Magnet-Klauber v4 (Autodesk Fusion 360 archive; units mm, degrees)
design "Gleitgestell"
Autodesk Fusion 360 part; units mm, degrees
(part 1 of 2)
sketch "Skizze1" plane through (0, 0, 0) normal (0, 0, 1) x (1, 0, 0)
  line L0 (0, 0) -> (18.25, 0) construction
  line L1 (18.25, 0) -> (30.25, 0)
  line L2 (30.25, 0) -> (30.25, 22)
  line L3 (30.25, 22) -> (18.25, 22)
  line L4 (18.25, 22) -> (18.25, 0)
  circle A0 centre (26.25, 14.5) radius 1.5
  line L5 (0, 25) -> (0, 0) construction
  line L6 (-18.25, 22) -> (-18.25, 0)
  line L7 (-18.25, 0) -> (-30.25, 0)
  line L8 (-30.25, 0) -> (-30.25, 22)
  circle A1 centre (-26.25, 14.5) radius 1.5
  line L9 (-30.25, 22) -> (-18.25, 22)
  dimension "d8" = 12
  dimension "d9" = 22
  dimension "d10" = 3
  dimension "d11" = 4
  dimension "d12" = 7.5
  dimension "d25" = 26.25
  constraint coincident L0.start L5.end
  constraint horizontal L0
  constraint horizontal L1
  constraint vertical L2
  constraint horizontal L3
  constraint vertical L4
  constraint vertical L5
  constraint symmetric L0.end L5 L6.end
  constraint symmetric L1.end L5 L7.end
  constraint symmetric L2.end L5 L8.end
  constraint symmetric L3.end L5 L6.start
  constraint symmetric A0 L5 A1
  measures "d8" distance of L0.end L1.end
  measures "d9" distance of L0.end L3.end
  measures "d10" diameter of A0
  measures "d11" distance of L2 A0.centre
  measures "d12" distance of L3 A0.centre
  measures "d25" distance of A0.centre L5
extrude "Extrusion1" add sketch "Skizze1" against normal blind 3 makes body 1 at (24.8054, 4.3459, 0) makes body 2 at (-24.8054, 4.3459, 0)
sketch "Skizze2" plane through (0, 0, -3) normal (0, 0, -1) x (1, 0, 0)
  circle A0 centre (-26.25, -14.5) radius 1.5
  line L0 (-30.25, 0) -> (-30.25, -22)
  line L1 (-30.25, -22) -> (-18.25, -22)
  line L2 (-18.25, -22) -> (-18.25, 0)
  line L3 (-18.25, 0) -> (-30.25, 0)
  circle A1 centre (26.25, -14.5) radius 1.5
  line L4 (18.25, 0) -> (30.25, 0)
  line L5 (30.25, 0) -> (30.25, -22)
  line L6 (30.25, -22) -> (18.25, -22)
  line L7 (18.25, -22) -> (18.25, 0)
  circle A2 centre (-26.25, -14.5) radius 1.5
  line L8 (-18.25, 0) -> (-30.25, 0)
  line L9 (-18.25, -22) -> (-18.25, 0)
  line L10 (-30.25, -22) -> (-18.25, -22)
  line L11 (-30.25, 0) -> (-30.25, -22)
  line L12 (-30.25, 1) -> (-18.25, 1)
  line L13 (-18.25, 1) -> (-18.25, -22)
  line L14 (-30.25, -22) -> (-30.25, 1)
  line L15 (0, 0) -> (0, -27) construction
  line L16 (18.25, -22) -> (30.25, -22)
  line L17 (30.25, 1) -> (18.25, 1)
  dimension "d27" = 1
  constraint horizontal L12
  constraint vertical L13
  constraint vertical L14
  constraint coincident L11 L12.start
  constraint coincident L15.start origin
  constraint vertical L15
  constraint symmetric L12.start L15 L17.start
  constraint symmetric L12.end L15 L17.end
  constraint symmetric L1.end L15 L6.end
  constraint symmetric L0.end L15 L5.end
  constraint coincident L1.end L2.start
  constraint coincident L0.end L1.start
  measures "d27" distance of L8 L12
extrude "Extrusion2" add sketch "Skizze2" along normal blind 29 contours A0 A2 | L0 L1 L2 L3 L8 L9 L10 L11 L13 L14 | A1 | L4 L5 L6 L7 L16 bodies 1 2
thread "Gewinde1" "ISO Metric profile 3.0 M3x0.5 6H" major diameter 3.086 minor diameter 2.529 pitch 0.5 angle 60 resizes the face on face at (-24.7519, 14.4252, -2) on face at (27.7481, 14.4252, -2) on bodies 1 2
sketch "Skizze3" plane through (30.25, 0, 0) normal (1, 0, 0) x (0, 1, 0)
  line L0 (22, 0) -> (0, 0)
  line L1 (0, 0) -> (0, -32)
  line L2 (0, -32) -> (22, -32)
  line L3 (22, -32) -> (22, 0)
  circle A0 centre (9.5, -22) radius 6.5
  dimension "d19" = 13
  dimension "d24" = 22
  dimension "d28" = 9.5
  measures "d19" diameter of A0
  measures "d24" distance of L0 A0.centre
  measures "d28" distance of L1 A0.centre
extrude "Extrusion3" cut sketch "Skizze3" against normal blind 93 contours A0 bodies 1 2

design "2020_T-Nut"
Autodesk Fusion 360 part; units mm, degrees
sketch "Skizze1" plane through (0, 0, 0) normal (1, 0, 0) x (0, 1, 0)
  line L0 (0, 0) -> (3.5, 0)
  line L1 (5, 1.5) -> (5, 3.3)
  line L2 (5, 3.3) -> (2.5, 3.3)
  line L3 (2.5, 3.3) -> (2.5, 5)
  line L4 (3.5, 0) -> (5, 1.5)
  line L5 (0, 5) -> (0, 0) construction
  line L6 (-5, 1.5) -> (-5, 3.3)
  line L7 (-5, 3.3) -> (-2.5, 3.3)
  line L8 (0, 0) -> (-3.5, 0)
  line L9 (-3.5, 0) -> (-5, 1.5)
  line L10 (-2.5, 3.3) -> (-2.5, 5)
  line L11 (-2.5, 5) -> (2.5, 5)
  point P0 (5, 0)
  point P1 (-5, 0)
  point P2 (0, 0)
  point P3 (0, 0)
  dimension "d1" = 5
  dimension "d3" = 2.5
  dimension "d4" = 3.3
  dimension "d5" = 1.5
  dimension "d6" = 1.5
  constraint coincident P3 P2
  constraint horizontal L0
  constraint perpendicular L0 L1
  constraint perpendicular L1 L2
  constraint perpendicular L2 L3
  constraint coincident P0 L0
  constraint coincident P0 L1
  constraint perpendicular L0 L5
  constraint symmetric P3 L5 P2
  constraint symmetric P0 L5 P1
  constraint symmetric L1.end L5 L6.end
  constraint symmetric L2.end L5 L7.end
  constraint symmetric L3.end L5 L10.end
  constraint symmetric L0.end L5 L8.end
  constraint symmetric L1.start L5 L6.start
  measures "d1" distance of P3 P0
  measures "d3" distance of L1.end L2.end
  measures "d4" distance of L0 L2
  measures "d5" distance of P0 L0.end
  measures "d6" distance of P0 L1.start
extrude "Extrusion1" add sketch "Skizze1" along normal blind 11.5
sketch "Skizze2" plane through (0, 0, 5) normal (0, 0, 1) x (-1, 0, 0)
  line L0 (0, 0) -> (0, 2.5)
  line L1 (0, 2.5) -> (-11.5, 2.5)
  line L2 (-11.5, -2.5) -> (0, -2.5)
  circle A0 centre (-5.75, 0) radius 2
  line L3 (-11.5, 2.5) -> (-11.5, 0)
  line L4 (0, -2.5) -> (0, 0)
  line L5 (0, 0) -> (-11.5, 0)
  line L6 (-11.5, 0) -> (-11.5, -2.5)
  dimension "d9" = 4
  measures "d9" diameter of A0
extrude "Extrusion2" cut sketch "Skizze2" against normal blind 5.5 contours A0 L5 | A0 L5
thread "Gewinde1" "ISO Metric profile 4.0 M4x0.7 6H" major diameter 4.1095 minor diameter 3.332 pitch 0.7 angle 60 resizes the face on face at (7.7401, 0.1991, 1.6667)

design "Riemen"
Autodesk Fusion 360 part; units mm, degrees
sketch "Skizze1" plane through (0, 0, 0) normal (0, 0, 1) x (1, 0, 0)
  line L0 (-200, 5) -> (0, 5)
  line L1 (0, -5) -> (-200, -5)
  line L2 (0, -6) -> (-200, -6)
  line L3 (-200, 6) -> (0, 6)
  line L4 (-200, 5) -> (-200, -5) construction
  arc A0 (-200, 6) -> (-200, -6) centre (-200, 0) ccw
  arc A1 (-200, 5) -> (-200, -5) centre (-200, 0) ccw
  line L5 (0, -10) -> (0, 7.5) construction
  circle A2 centre (-1, -5) radius 0.5
  circle A3 centre (-3.0202, -5) radius 0.5
  circle A4 centre (-5.0404, -5) radius 0.5
  circle A5 centre (-7.0606, -5) radius 0.5
  circle A6 centre (-9.0808, -5) radius 0.5
  circle A7 centre (-11.101, -5) radius 0.5
  circle A8 centre (-13.1212, -5) radius 0.5
  circle A9 centre (-15.1414, -5) radius 0.5
  circle A10 centre (-17.1616, -5) radius 0.5
  circle A11 centre (-19.1818, -5) radius 0.5
  circle A12 centre (-21.202, -5) radius 0.5
  circle A13 centre (-23.2222, -5) radius 0.5
  circle A14 centre (-25.2424, -5) radius 0.5
  circle A15 centre (-27.2626, -5) radius 0.5
  circle A16 centre (-29.2828, -5) radius 0.5
  circle A17 centre (-31.303, -5) radius 0.5
  circle A18 centre (-33.3232, -5) radius 0.5
  circle A19 centre (-35.3434, -5) radius 0.5
  circle A20 centre (-37.3636, -5) radius 0.5
  circle A21 centre (-39.3838, -5) radius 0.5
  circle A22 centre (-41.404, -5) radius 0.5
  circle A23 centre (-43.4242, -5) radius 0.5
  circle A24 centre (-45.4444, -5) radius 0.5
  circle A25 centre (-47.4646, -5) radius 0.5
  circle A26 centre (-49.4848, -5) radius 0.5
  circle A27 centre (-51.5051, -5) radius 0.5
  circle A28 centre (-53.5253, -5) radius 0.5
  circle A29 centre (-55.5455, -5) radius 0.5
  circle A30 centre (-57.5657, -5) radius 0.5
  circle A31 centre (-59.5859, -5) radius 0.5
  circle A32 centre (-61.6061, -5) radius 0.5
  circle A33 centre (-63.6263, -5) radius 0.5
  circle A34 centre (-65.6465, -5) radius 0.5
  circle A35 centre (-67.6667, -5) radius 0.5
  circle A36 centre (-69.6869, -5) radius 0.5
  circle A37 centre (-71.7071, -5) radius 0.5
  circle A38 centre (-73.7273, -5) radius 0.5
  circle A39 centre (-75.7475, -5) radius 0.5
  circle A40 centre (-77.7677, -5) radius 0.5
  circle A41 centre (-79.7879, -5) radius 0.5
  circle A42 centre (-81.8081, -5) radius 0.5
  circle A43 centre (-83.8283, -5) radius 0.5
  circle A44 centre (-85.8485, -5) radius 0.5
  circle A45 centre (-87.8687, -5) radius 0.5
  circle A46 centre (-89.8889, -5) radius 0.5
  circle A47 centre (-91.9091, -5) radius 0.5
  circle A48 centre (-93.9293, -5) radius 0.5
  circle A49 centre (-95.9495, -5) radius 0.5
  circle A50 centre (-97.9697, -5) radius 0.5
  circle A51 centre (-99.9899, -5) radius 0.5
  circle A52 centre (-102.0101, -5) radius 0.5
  circle A53 centre (-104.0303, -5) radius 0.5
  circle A54 centre (-106.0505, -5) radius 0.5
  circle A55 centre (-108.0707, -5) radius 0.5
  circle A56 centre (-110.0909, -5) radius 0.5
  circle A57 centre (-112.1111, -5) radius 0.5
  circle A58 centre (-114.1313, -5) radius 0.5
  circle A59 centre (-116.1515, -5) radius 0.5
  circle A60 centre (-118.1717, -5) radius 0.5
  circle A61 centre (-120.1919, -5) radius 0.5
  circle A62 centre (-122.2121, -5) radius 0.5
  circle A63 centre (-124.2323, -5) radius 0.5
  circle A64 centre (-126.2525, -5) radius 0.5
  circle A65 centre (-128.2727, -5) radius 0.5
  circle A66 centre (-130.2929, -5) radius 0.5
  circle A67 centre (-132.3131, -5) radius 0.5
  circle A68 centre (-134.3333, -5) radius 0.5
  circle A69 centre (-136.3535, -5) radius 0.5
  circle A70 centre (-138.3737, -5) radius 0.5
  circle A71 centre (-140.3939, -5) radius 0.5
  circle A72 centre (-142.4141, -5) radius 0.5
  circle A73 centre (-144.4343, -5) radius 0.5
  circle A74 centre (-146.4545, -5) radius 0.5
  circle A75 centre (-148.4747, -5) radius 0.5
  circle A76 centre (-150.4949, -5) radius 0.5
  circle A77 centre (-152.5152, -5) radius 0.5
  circle A78 centre (-154.5354, -5) radius 0.5
  circle A79 centre (-156.5556, -5) radius 0.5
  circle A80 centre (-158.5758, -5) radius 0.5
  circle A81 centre (-160.596, -5) radius 0.5
  circle A82 centre (-162.6162, -5) radius 0.5
  circle A83 centre (-164.6364, -5) radius 0.5
  circle A84 centre (-166.6566, -5) radius 0.5
  circle A85 centre (-168.6768, -5) radius 0.5
  circle A86 centre (-170.697, -5) radius 0.5
  circle A87 centre (-172.7172, -5) radius 0.5
  circle A88 centre (-174.7374, -5) radius 0.5
  circle A89 centre (-176.7576, -5) radius 0.5
  circle A90 centre (-178.7778, -5) radius 0.5
  circle A91 centre (-180.798, -5) radius 0.5
  circle A92 centre (-182.8182, -5) radius 0.5
  circle A93 centre (-184.8384, -5) radius 0.5
  circle A94 centre (-186.8586, -5) radius 0.5
  circle A95 centre (-188.8788, -5) radius 0.5
  circle A96 centre (-190.899, -5) radius 0.5
  circle A97 centre (-192.9192, -5) radius 0.5
  circle A98 centre (-194.9394, -5) radius 0.5
  circle A99 centre (-196.9596, -5) radius 0.5
  circle A100 centre (-198.9798, -5) radius 0.5
  circle A101 centre (-205, 0) radius 0.5
  circle A102 centre (-201.5035, 4.7686) radius 0.5
  circle A103 centre (-203.324, 3.7351) radius 0.5
  circle A104 centre (-204.5618, 2.047) radius 0.5
  circle A105 centre (-204.5618, -2.047) radius 0.5
  circle A106 centre (-203.324, -3.7351) radius 0.5
  circle A107 centre (-201.5035, -4.7686) radius 0.5
  circle A108 centre (-1, 5) radius 0.5
  circle A109 centre (-3.0204, 5) radius 0.5
  circle A110 centre (-5.0408, 5) radius 0.5
  circle A111 centre (-7.0612, 5) radius 0.5
  circle A112 centre (-9.0816, 5) radius 0.5
  circle A113 centre (-11.102, 5) radius 0.5
  circle A114 centre (-13.1224, 5) radius 0.5
  circle A115 centre (-15.1429, 5) radius 0.5
  circle A116 centre (-17.1633, 5) radius 0.5
  circle A117 centre (-19.1837, 5) radius 0.5
  circle A118 centre (-21.2041, 5) radius 0.5
  circle A119 centre (-23.2245, 5) radius 0.5
  circle A120 centre (-25.2449, 5) radius 0.5
  circle A121 centre (-27.2653, 5) radius 0.5
  circle A122 centre (-29.2857, 5) radius 0.5
  circle A123 centre (-31.3061, 5) radius 0.5
  circle A124 centre (-33.3265, 5) radius 0.5
  circle A125 centre (-35.3469, 5) radius 0.5
  circle A126 centre (-37.3673, 5) radius 0.5
  circle A127 centre (-39.3878, 5) radius 0.5
  circle A128 centre (-41.4082, 5) radius 0.5
  circle A129 centre (-43.4286, 5) radius 0.5
  circle A130 centre (-45.449, 5) radius 0.5
  circle A131 centre (-47.4694, 5) radius 0.5
  circle A132 centre (-49.4898, 5) radius 0.5
  circle A133 centre (-51.5102, 5) radius 0.5
  circle A134 centre (-53.5306, 5) radius 0.5
  circle A135 centre (-55.551, 5) radius 0.5
  circle A136 centre (-57.5714, 5) radius 0.5
  circle A137 centre (-59.5918, 5) radius 0.5
  circle A138 centre (-61.6122, 5) radius 0.5
  circle A139 centre (-63.6327, 5) radius 0.5
  circle A140 centre (-65.6531, 5) radius 0.5
  circle A141 centre (-67.6735, 5) radius 0.5
  circle A142 centre (-69.6939, 5) radius 0.5
  circle A143 centre (-71.7143, 5) radius 0.5
  circle A144 centre (-73.7347, 5) radius 0.5
  circle A145 centre (-75.7551, 5) radius 0.5
  circle A146 centre (-77.7755, 5) radius 0.5
  circle A147 centre (-79.7959, 5) radius 0.5
  circle A148 centre (-81.8163, 5) radius 0.5
  circle A149 centre (-83.8367, 5) radius 0.5
  circle A150 centre (-85.8571, 5) radius 0.5
  circle A151 centre (-87.8776, 5) radius 0.5
  circle A152 centre (-89.898, 5) radius 0.5
  circle A153 centre (-91.9184, 5) radius 0.5
  circle A154 centre (-93.9388, 5) radius 0.5
  circle A155 centre (-95.9592, 5) radius 0.5
  circle A156 centre (-97.9796, 5) radius 0.5
  circle A157 centre (-100, 5) radius 0.5
  circle A158 centre (-102.0204, 5) radius 0.5
  circle A159 centre (-104.0408, 5) radius 0.5
  circle A160 centre (-106.0612, 5) radius 0.5
  circle A161 centre (-108.0816, 5) radius 0.5
  circle A162 centre (-110.102, 5) radius 0.5
  circle A163 centre (-112.1224, 5) radius 0.5
  circle A164 centre (-114.1429, 5) radius 0.5
  circle A165 centre (-116.1633, 5) radius 0.5
  circle A166 centre (-118.1837, 5) radius 0.5
  circle A167 centre (-120.2041, 5) radius 0.5
  circle A168 centre (-122.2245, 5) radius 0.5
  circle A169 centre (-124.2449, 5) radius 0.5
  circle A170 centre (-126.2653, 5) radius 0.5
  circle A171 centre (-128.2857, 5) radius 0.5
  circle A172 centre (-130.3061, 5) radius 0.5
  circle A173 centre (-132.3265, 5) radius 0.5
  circle A174 centre (-134.3469, 5) radius 0.5
  circle A175 centre (-136.3673, 5) radius 0.5
  circle A176 centre (-138.3878, 5) radius 0.5
  circle A177 centre (-140.4082, 5) radius 0.5
  circle A178 centre (-142.4286, 5) radius 0.5
  circle A179 centre (-144.449, 5) radius 0.5
  circle A180 centre (-146.4694, 5) radius 0.5
  circle A181 centre (-148.4898, 5) radius 0.5
  circle A182 centre (-150.5102, 5) radius 0.5
  circle A183 centre (-152.5306, 5) radius 0.5
  circle A184 centre (-154.551, 5) radius 0.5
  circle A185 centre (-156.5714, 5) radius 0.5
  circle A186 centre (-158.5918, 5) radius 0.5
  circle A187 centre (-160.6122, 5) radius 0.5
  circle A188 centre (-162.6327, 5) radius 0.5
  circle A189 centre (-164.6531, 5) radius 0.5
  circle A190 centre (-166.6735, 5) radius 0.5
  circle A191 centre (-168.6939, 5) radius 0.5
  circle A192 centre (-170.7143, 5) radius 0.5
  circle A193 centre (-172.7347, 5) radius 0.5
  circle A194 centre (-174.7551, 5) radius 0.5
  circle A195 centre (-176.7755, 5) radius 0.5
  circle A196 centre (-178.7959, 5) radius 0.5
  circle A197 centre (-180.8163, 5) radius 0.5
  circle A198 centre (-182.8367, 5) radius 0.5
  circle A199 centre (-184.8571, 5) radius 0.5
  circle A200 centre (-186.8776, 5) radius 0.5
  circle A201 centre (-188.898, 5) radius 0.5
  circle A202 centre (-190.9184, 5) radius 0.5
  circle A203 centre (-192.9388, 5) radius 0.5
  circle A204 centre (-194.9592, 5) radius 0.5
  circle A205 centre (-196.9796, 5) radius 0.5
  circle A206 centre (-199, 5) radius 0.5
  line L6 (200, 5) -> (0, 5)
  circle A207 centre (13.1224, 5) radius 0.5
  circle A208 centre (25.2449, 5) radius 0.5
  circle A209 centre (67.6735, 5) radius 0.5
  circle A210 centre (89.8889, -5) radius 0.5
  circle A211 centre (158.5918, 5) radius 0.5
  circle A212 centre (118.1717, -5) radius 0.5
  circle A213 centre (73.7347, 5) radius 0.5
  circle A214 centre (19.1818, -5) radius 0.5
  circle A215 centre (29.2857, 5) radius 0.5
  circle A216 centre (5.0408, 5) radius 0.5
  circle A217 centre (162.6327, 5) radius 0.5
  circle A218 centre (128.2857, 5) radius 0.5
  circle A219 centre (43.4242, -5) radius 0.5
  circle A220 centre (116.1633, 5) radius 0.5
  circle A221 centre (23.2222, -5) radius 0.5
  circle A222 centre (75.7475, -5) radius 0.5
  circle A223 centre (172.7172, -5) radius 0.5
  circle A224 centre (53.5306, 5) radius 0.5
  circle A225 centre (31.3061, 5) radius 0.5
  circle A226 centre (95.9495, -5) radius 0.5
  circle A227 centre (87.8776, 5) radius 0.5
  line L7 (200, 6) -> (0, 6)
  line L8 (0, -5) -> (200, -5)
  line L9 (0, -6) -> (200, -6)
  circle A228 centre (19.1837, 5) radius 0.5
  circle A229 centre (168.6939, 5) radius 0.5
  circle A230 centre (102.0101, -5) radius 0.5
  circle A231 centre (71.7071, -5) radius 0.5
  circle A232 centre (63.6263, -5) radius 0.5
  circle A233 centre (114.1313, -5) radius 0.5
  circle A234 centre (51.5051, -5) radius 0.5
  circle A235 centre (27.2653, 5) radius 0.5
  circle A236 centre (106.0612, 5) radius 0.5
  circle A237 centre (164.6364, -5) radius 0.5
  circle A238 centre (7.0606, -5) radius 0.5
  circle A239 centre (81.8163, 5) radius 0.5
  circle A240 centre (21.2041, 5) radius 0.5
  circle A241 centre (170.697, -5) radius 0.5
  circle A242 centre (79.7879, -5) radius 0.5
  circle A243 centre (49.4848, -5) radius 0.5
  circle A244 centre (67.6667, -5) radius 0.5
  circle A245 centre (23.2245, 5) radius 0.5
  circle A246 centre (122.2121, -5) radius 0.5
  circle A247 centre (160.596, -5) radius 0.5
  circle A248 centre (126.2525, -5) radius 0.5
  circle A249 centre (174.7551, 5) radius 0.5
  circle A250 centre (122.2245, 5) radius 0.5
  circle A251 centre (162.6162, -5) radius 0.5
  circle A252 centre (37.3673, 5) radius 0.5
  circle A253 centre (97.9796, 5) radius 0.5
  circle A254 centre (1, 5) radius 0.5
  circle A255 centre (17.1616, -5) radius 0.5
  circle A256 centre (33.3265, 5) radius 0.5
  circle A257 centre (104.0408, 5) radius 0.5
  circle A258 centre (95.9592, 5) radius 0.5
  circle A259 centre (65.6465, -5) radius 0.5
  circle A260 centre (172.7347, 5) radius 0.5
  circle A261 centre (13.1212, -5) radius 0.5
  circle A262 centre (3.0202, -5) radius 0.5
  circle A263 centre (93.9293, -5) radius 0.5
  circle A264 centre (75.7551, 5) radius 0.5
  circle A265 centre (63.6327, 5) radius 0.5
  circle A266 centre (180.798, -5) radius 0.5
  circle A267 centre (15.1414, -5) radius 0.5
  circle A268 centre (1, -5) radius 0.5
  circle A269 centre (126.2653, 5) radius 0.5
  circle A270 centre (57.5714, 5) radius 0.5
  circle A271 centre (108.0816, 5) radius 0.5
  circle A272 centre (49.4898, 5) radius 0.5
  circle A273 centre (35.3434, -5) radius 0.5
  circle A274 centre (83.8367, 5) radius 0.5
  circle A275 centre (124.2449, 5) radius 0.5
  circle A276 centre (85.8485, -5) radius 0.5
  circle A277 centre (166.6566, -5) radius 0.5
  circle A278 centre (69.6869, -5) radius 0.5
  circle A279 centre (45.449, 5) radius 0.5
  circle A280 centre (53.5253, -5) radius 0.5
  circle A281 centre (47.4646, -5) radius 0.5
  circle A282 centre (65.6531, 5) radius 0.5
  circle A283 centre (158.5758, -5) radius 0.5
  circle A284 centre (91.9184, 5) radius 0.5
  circle A285 centre (118.1837, 5) radius 0.5
  circle A286 centre (178.7959, 5) radius 0.5
  circle A287 centre (102.0204, 5) radius 0.5
  circle A288 centre (128.2727, -5) radius 0.5
  circle A289 centre (168.6768, -5) radius 0.5
  circle A290 centre (39.3838, -5) radius 0.5
  circle A291 centre (17.1633, 5) radius 0.5
  circle A292 centre (124.2323, -5) radius 0.5
  circle A293 centre (27.2626, -5) radius 0.5
  circle A294 centre (184.8571, 5) radius 0.5
  circle A295 centre (104.0303, -5) radius 0.5
  circle A296 centre (110.102, 5) radius 0.5
  circle A297 centre (99.9899, -5) radius 0.5
  circle A298 centre (156.5556, -5) radius 0.5
  circle A299 centre (41.4082, 5) radius 0.5
  circle A300 centre (97.9697, -5) radius 0.5
  circle A301 centre (110.0909, -5) radius 0.5
  circle A302 centre (73.7273, -5) radius 0.5
  circle A303 centre (37.3636, -5) radius 0.5
  circle A304 centre (116.1515, -5) radius 0.5
  circle A305 centre (5.0404, -5) radius 0.5
  circle A306 centre (45.4444, -5) radius 0.5
  circle A307 centre (77.7755, 5) radius 0.5
  circle A308 centre (55.5455, -5) radius 0.5
  circle A309 centre (39.3878, 5) radius 0.5
  circle A310 centre (11.102, 5) radius 0.5
  circle A311 centre (174.7374, -5) radius 0.5
  circle A312 centre (176.7755, 5) radius 0.5
  circle A313 centre (9.0816, 5) radius 0.5
  circle A314 centre (59.5859, -5) radius 0.5
  circle A315 centre (57.5657, -5) radius 0.5
  circle A316 centre (112.1111, -5) radius 0.5
  circle A317 centre (156.5714, 5) radius 0.5
  circle A318 centre (9.0808, -5) radius 0.5
  circle A319 centre (120.1919, -5) radius 0.5
  circle A320 centre (61.6122, 5) radius 0.5
  circle A321 centre (43.4286, 5) radius 0.5
  circle A322 centre (15.1429, 5) radius 0.5
  circle A323 centre (11.101, -5) radius 0.5
  circle A324 centre (120.2041, 5) radius 0.5
  circle A325 centre (91.9091, -5) radius 0.5
  circle A326 centre (25.2424, -5) radius 0.5
  circle A327 centre (93.9388, 5) radius 0.5
  circle A328 centre (178.7778, -5) radius 0.5
  circle A329 centre (59.5918, 5) radius 0.5
  circle A330 centre (69.6939, 5) radius 0.5
  circle A331 centre (21.202, -5) radius 0.5
  circle A332 centre (176.7576, -5) radius 0.5
  circle A333 centre (79.7959, 5) radius 0.5
  circle A334 centre (170.7143, 5) radius 0.5
  circle A335 centre (7.0612, 5) radius 0.5
  circle A336 centre (89.898, 5) radius 0.5
  circle A337 centre (61.6061, -5) radius 0.5
  circle A338 centre (29.2828, -5) radius 0.5
  circle A339 centre (33.3232, -5) radius 0.5
  circle A340 centre (3.0204, 5) radius 0.5
  circle A341 centre (114.1429, 5) radius 0.5
  circle A342 centre (203.324, 3.7351) radius 0.5
  circle A343 centre (130.2929, -5) radius 0.5
  circle A344 centre (190.9184, 5) radius 0.5
  circle A345 centre (136.3535, -5) radius 0.5
  circle A346 centre (134.3469, 5) radius 0.5
  circle A347 centre (148.4747, -5) radius 0.5
  circle A348 centre (196.9796, 5) radius 0.5
  circle A349 centre (194.9592, 5) radius 0.5
  circle A350 centre (152.5306, 5) radius 0.5
  circle A351 centre (132.3265, 5) radius 0.5
  circle A352 centre (199, 5) radius 0.5
  circle A353 centre (152.5152, -5) radius 0.5
  circle A354 centre (148.4898, 5) radius 0.5
  circle A355 centre (204.5618, -2.047) radius 0.5
  circle A356 centre (186.8586, -5) radius 0.5
  line L10 (200, 5) -> (200, -5) construction
  circle A357 centre (204.5618, 2.047) radius 0.5
  circle A358 centre (130.3061, 5) radius 0.5
  arc A359 (200, -5) -> (200, 5) centre (200, 0) ccw
  circle A360 centre (154.551, 5) radius 0.5
  circle A361 centre (188.8788, -5) radius 0.5
  circle A362 centre (188.898, 5) radius 0.5
  circle A363 centre (146.4694, 5) radius 0.5
  circle A364 centre (154.5354, -5) radius 0.5
  circle A365 centre (150.4949, -5) radius 0.5
  circle A366 centre (180.8163, 5) radius 0.5
  circle A367 centre (134.3333, -5) radius 0.5
  circle A368 centre (146.4545, -5) radius 0.5
  circle A369 centre (85.8571, 5) radius 0.5
  circle A370 centre (192.9388, 5) radius 0.5
  circle A371 centre (194.9394, -5) radius 0.5
  circle A372 centre (108.0707, -5) radius 0.5
  circle A373 centre (77.7677, -5) radius 0.5
  circle A374 centre (164.6531, 5) radius 0.5
  circle A375 centre (47.4694, 5) radius 0.5
  circle A376 centre (198.9798, -5) radius 0.5
  circle A377 centre (142.4286, 5) radius 0.5
  circle A378 centre (140.4082, 5) radius 0.5
  circle A379 centre (184.8384, -5) radius 0.5
  circle A380 centre (190.899, -5) radius 0.5
  circle A381 centre (138.3737, -5) radius 0.5
  circle A382 centre (81.8081, -5) radius 0.5
  circle A383 centre (182.8182, -5) radius 0.5
  circle A384 centre (136.3673, 5) radius 0.5
  arc A385 (200, -6) -> (200, 6) centre (200, 0) ccw
  circle A386 centre (201.5035, -4.7686) radius 0.5
  circle A387 centre (138.3878, 5) radius 0.5
  circle A388 centre (203.324, -3.7351) radius 0.5
  circle A389 centre (205, 0) radius 0.5
  circle A390 centre (140.3939, -5) radius 0.5
  circle A391 centre (182.8367, 5) radius 0.5
  circle A392 centre (31.303, -5) radius 0.5
  circle A393 centre (35.3469, 5) radius 0.5
  circle A394 centre (160.6122, 5) radius 0.5
  circle A395 centre (192.9192, -5) radius 0.5
  circle A396 centre (150.5102, 5) radius 0.5
  circle A397 centre (132.3131, -5) radius 0.5
  circle A398 centre (186.8776, 5) radius 0.5
  circle A399 centre (112.1224, 5) radius 0.5
  circle A400 centre (166.6735, 5) radius 0.5
  circle A401 centre (144.449, 5) radius 0.5
  circle A402 centre (144.4343, -5) radius 0.5
  circle A403 centre (55.551, 5) radius 0.5
  circle A404 centre (41.404, -5) radius 0.5
  circle A405 centre (196.9596, -5) radius 0.5
  circle A406 centre (71.7143, 5) radius 0.5
  circle A407 centre (142.4141, -5) radius 0.5
  circle A408 centre (87.8687, -5) radius 0.5
  circle A409 centre (100, 5) radius 0.5
  circle A410 centre (51.5102, 5) radius 0.5
  circle A411 centre (106.0505, -5) radius 0.5
  circle A412 centre (83.8283, -5) radius 0.5
  circle A413 centre (201.5035, 4.7686) radius 0.5
  point P0 (0, -10)
  point P1 (0, 7.5)
  dimension "d3" = 10
  dimension "d4" = 5
  dimension "d6" = 1
  dimension "d7" = 1
  dimension "d10" = -200
  dimension "d11" = 0
  dimension "d14" = 200
  dimension "d17" = 1
  dimension "d19" = 145
  dimension "d20" = 1
  dimension "d21" = 1
  dimension "d24" = -198
  dimension "d25" = -200
  constraint horizontal L0
  constraint horizontal L1
  constraint parallel L1 L2
  constraint parallel L0 L3
  constraint perpendicular L2 L4
  constraint tangent L0 A1
  constraint concentric A0 A1
  constraint perpendicular L3 L5
  constraint coincident L5 L2.start
  constraint coincident L5 L1.start
  constraint coincident L5 L0.end
  constraint coincident L5 L3.end
  constraint coincident L1 A2.centre
  constraint midpoint A1 A101.centre
  constraint coincident L4 A0.centre
  constraint coincident L0 A108.centre
  constraint symmetric L0.start L5 L6.start
  constraint symmetric L1.end L5 L8.end
  constraint symmetric L3.start L5 L7.start
  constraint symmetric L2.end L5 L9.end
  constraint symmetric A0 L5 A385
  constraint symmetric A1 L5 A359
  constraint symmetric P0 L5 L5.start
  constraint symmetric P1 L5 L5.end
  constraint symmetric L5 L2.start L9.start
  constraint symmetric L5 L1.start L8.start
  constraint symmetric L5 L0.end L6.end
  constraint symmetric L5 L3.end L7.end
  constraint symmetric L5 A2 A268
  constraint symmetric L5 A3 A262
  constraint symmetric L5 A4 A305
  constraint symmetric L5 A5 A238
  constraint symmetric L5 A6 A318
  constraint symmetric L5 A7 A323
  constraint symmetric L5 A8 A261
  constraint symmetric L5 A9 A267
  constraint symmetric L5 A10 A255
  constraint symmetric L5 A11 A214
  constraint symmetric L5 A12 A331
  constraint symmetric L5 A13 A221
  constraint symmetric L5 A14 A326
  constraint symmetric L5 A15 A293
  constraint symmetric L5 A16 A338
  constraint symmetric L5 A17 A392
  constraint symmetric L5 A18 A339
  constraint symmetric L5 A19 A273
  constraint symmetric L5 A20 A303
  constraint symmetric L5 A21 A290
  constraint symmetric L5 A22 A404
  constraint symmetric L5 A23 A219
  constraint symmetric L5 A24 A306
  constraint symmetric L5 A25 A281
  constraint symmetric L5 A26 A243
  constraint symmetric L5 A27 A234
  constraint symmetric L5 A28 A280
  constraint symmetric L5 A29 A308
  constraint symmetric L5 A30 A315
  constraint symmetric L5 A31 A314
  constraint symmetric L5 A32 A337
  constraint symmetric L5 A33 A232
  constraint symmetric L5 A34 A259
  constraint symmetric L5 A35 A244
  constraint symmetric L5 A36 A278
  constraint symmetric L5 A37 A231
  constraint symmetric L5 A38 A302
  constraint symmetric L5 A39 A222
  constraint symmetric L5 A40 A373
  constraint symmetric L5 A41 A242
  constraint symmetric L5 A42 A382
  constraint symmetric L5 A43 A412
  constraint symmetric L5 A44 A276
  constraint symmetric L5 A45 A408
  constraint symmetric L5 A46 A210
  constraint symmetric L5 A47 A325
  constraint symmetric L5 A48 A263
  constraint symmetric L5 A49 A226
  constraint symmetric L5 A50 A300
  constraint symmetric L5 A51 A297
  constraint symmetric L5 A52 A230
  constraint symmetric L5 A53 A295
  constraint symmetric L5 A54 A411
  constraint symmetric L5 A55 A372
  constraint symmetric L5 A56 A301
  constraint symmetric L5 A57 A316
  constraint symmetric L5 A58 A233
  constraint symmetric L5 A59 A304
  constraint symmetric L5 A60 A212
  constraint symmetric L5 A61 A319
  constraint symmetric L5 A62 A246
  constraint symmetric L5 A63 A292
  constraint symmetric L5 A64 A248
  constraint symmetric L5 A65 A288
  constraint symmetric L5 A66 A343
  constraint symmetric L5 A67 A397
  constraint symmetric L5 A68 A367
  constraint symmetric L5 A69 A345
  constraint symmetric L5 A70 A381
  constraint symmetric L5 A71 A390
  constraint symmetric L5 A72 A407
  constraint symmetric L5 A73 A402
  constraint symmetric L5 A74 A368
  constraint symmetric L5 A75 A347
  constraint symmetric L5 A76 A365
  constraint symmetric L5 A77 A353
  constraint symmetric L5 A78 A364
  constraint symmetric L5 A79 A298
  constraint symmetric L5 A80 A283
  constraint symmetric L5 A81 A247
  constraint symmetric L5 A82 A251
  constraint symmetric L5 A83 A237
  constraint symmetric L5 A84 A277
  constraint symmetric L5 A85 A289
  constraint symmetric L5 A86 A241
  constraint symmetric L5 A87 A223
  constraint symmetric L5 A88 A311
  constraint symmetric L5 A89 A332
  constraint symmetric L5 A90 A328
  constraint symmetric L5 A91 A266
  constraint symmetric L5 A92 A383
  constraint symmetric L5 A93 A379
  constraint symmetric L5 A94 A356
  constraint symmetric L5 A95 A361
  constraint symmetric L5 A96 A380
  constraint symmetric L5 A97 A395
  constraint symmetric L5 A98 A371
  constraint symmetric L5 A99 A405
  constraint symmetric L5 A100 A376
  constraint symmetric L5 A101 A389
  constraint symmetric L5 A102 A413
  constraint symmetric L5 A103 A342
  constraint symmetric L5 A104 A357
  constraint symmetric L5 A105 A355
  constraint symmetric L5 A106 A388
  constraint symmetric L5 A107 A386
  constraint symmetric L5 A108 A254
  constraint symmetric L5 A109 A340
  constraint symmetric L5 A110 A216
  constraint symmetric L5 A111 A335
  constraint symmetric L5 A112 A313
  constraint symmetric L5 A113 A310
  constraint symmetric L5 A114 A207
  constraint symmetric L5 A115 A322
  constraint symmetric L5 A116 A291
  constraint symmetric L5 A117 A228
  constraint symmetric L5 A118 A240
  constraint symmetric L5 A119 A245
  constraint symmetric L5 A120 A208
  constraint symmetric L5 A121 A235
  constraint symmetric L5 A122 A215
  constraint symmetric L5 A123 A225
  constraint symmetric L5 A124 A256
  constraint symmetric L5 A125 A393
  constraint symmetric L5 A126 A252
  constraint symmetric L5 A127 A309
  constraint symmetric L5 A128 A299
  constraint symmetric L5 A129 A321
  constraint symmetric L5 A130 A279
  constraint symmetric L5 A131 A375
  constraint symmetric L5 A132 A272
  constraint symmetric L5 A133 A410
  constraint symmetric L5 A134 A224
  constraint symmetric L5 A135 A403
  constraint symmetric L5 A136 A270
  constraint symmetric L5 A137 A329
  constraint symmetric L5 A138 A320
  constraint symmetric L5 A139 A265
  constraint symmetric L5 A140 A282
  constraint symmetric L5 A141 A209
  constraint symmetric L5 A142 A330
  constraint symmetric L5 A143 A406
  constraint symmetric L5 A144 A213
  constraint symmetric L5 A145 A264
  constraint symmetric L5 A146 A307
  constraint symmetric L5 A147 A333
  constraint symmetric L5 A148 A239
  constraint symmetric L5 A149 A274
  constraint symmetric L5 A150 A369
  constraint symmetric L5 A151 A227
  constraint symmetric L5 A152 A336
  constraint symmetric L5 A153 A284
  constraint symmetric L5 A154 A327
  constraint symmetric L5 A155 A258
  constraint symmetric L5 A156 A253
  constraint symmetric L5 A157 A409
  constraint symmetric L5 A158 A287
  constraint symmetric L5 A159 A257
  constraint symmetric L5 A160 A236
  constraint symmetric L5 A161 A271
  constraint symmetric L5 A162 A296
  constraint symmetric L5 A163 A399
  constraint symmetric L5 A164 A341
  constraint symmetric L5 A165 A220
  constraint symmetric L5 A166 A285
  constraint symmetric L5 A167 A324
  constraint symmetric L5 A168 A250
  constraint symmetric L5 A169 A275
  constraint symmetric L5 A170 A269
  constraint symmetric L5 A171 A218
  constraint symmetric L5 A172 A358
  constraint symmetric L5 A173 A351
  constraint symmetric L5 A174 A346
  constraint symmetric L5 A175 A384
  constraint symmetric L5 A176 A387
  constraint symmetric L5 A177 A378
  constraint symmetric L5 A178 A377
  constraint symmetric L5 A179 A401
  constraint symmetric L5 A180 A363
  constraint symmetric L5 A181 A354
  constraint symmetric L5 A182 A396
  constraint symmetric L5 A183 A350
  constraint symmetric L5 A184 A360
  constraint symmetric L5 A185 A317
  constraint symmetric L5 A186 A211
  constraint symmetric L5 A187 A394
  constraint symmetric L5 A188 A217
  constraint symmetric L5 A189 A374
  constraint symmetric L5 A190 A400
  constraint symmetric L5 A191 A229
  constraint symmetric L5 A192 A334
  constraint symmetric L5 A193 A260
  constraint symmetric L5 A194 A249
  constraint symmetric L5 A195 A312
  constraint symmetric L5 A196 A286
  constraint symmetric L5 A197 A366
  constraint symmetric L5 A198 A391
  constraint symmetric L5 A199 A294
  constraint symmetric L5 A200 A398
  constraint symmetric L5 A201 A362
  constraint symmetric L5 A202 A344
  constraint symmetric L5 A203 A370
  constraint symmetric L5 A204 A349
  constraint symmetric L5 A205 A348
  constraint symmetric L5 A206 A352
  measures "d3" distance of L0 L1
  measures "d4" distance of origin L0
  measures "d6" diameter of A2
  measures "d7" distance of L1.start A2.centre
  measures "d14" distance of origin L4
  measures "d17" diameter of A101
  measures "d20" diameter of A108
  measures "d21" distance of L0.end A108.centre
extrude "Extrusion1" add sketch "Skizze1" along normal blind 10

design "M4x6_Rundkopf+"
Autodesk Fusion 360 part; units mm, degrees
sketch "Skizze1" plane through (0, 0, 0) normal (0, 0, 1) x (1, 0, 0)
  circle A0 centre (0, 0) radius 4
  dimension "d1" = 8
  constraint coincident A0.centre origin
  measures "d1" diameter of A0
extrude "Extrusion1" add sketch "Skizze1" along normal blind 3
sketch "Skizze2" plane through (0, 0, 3) normal (0, 0, 1) x (-1, 0, 0)
  circle A0 centre (0, 0) radius 4
  line L0 (1.125, -0.625) -> (-1.125, -0.625)
  line L1 (-1.125, -0.625) -> (-1.125, 0.625)
  line L2 (-1.125, 0.625) -> (1.125, 0.625)
  line L3 (1.125, 0.625) -> (1.125, -0.625)
  line L4 (0.625, -1.125) -> (-0.625, -1.125)
  line L5 (-0.625, -1.125) -> (-0.625, 1.125)
  line L6 (-0.625, 1.125) -> (0.625, 1.125)
  line L7 (0.625, 1.125) -> (0.625, -1.125)
  dimension "d11" = 2.25
  dimension "d12" = 1.25
  dimension "d13" = 0.625
  dimension "d14" = 1.125
  dimension "d15" = 2.25
  dimension "d16" = 1.125
  dimension "d17" = 0.625
  dimension "d18" = 1.25
  constraint horizontal L0
  constraint vertical L1
  constraint horizontal L2
  constraint vertical L3
  constraint horizontal L4
  constraint vertical L5
  constraint horizontal L6
  constraint vertical L7
  measures "d11" distance of L0.start L0.end
  measures "d12" distance of L0.start L2.end
  measures "d13" distance of A0.centre L0
  measures "d14" distance of A0.centre L3
  measures "d15" distance of L4.end L5.end
  measures "d16" distance of A0.centre L4
  measures "d17" distance of A0.centre L5
  measures "d18" distance of L4.start L4.end
extrude "Extrusion2" cut sketch "Skizze2" against normal blind 1.2 contours L0 L2 L3 L7 | L0 L4 L5 L7 | L0 L2 L5 L7 | L0 L1 L2 L5 | L2 L5 L6 L7
chamfer "Fase3" distance 1.2 angle 45 4 edges at (0, 1.125, 3) (-1.125, 0, 3) (0, -1.125, 3) (1.125, 0, 3)
fillet "Abrundung1" radius 0.5 1 edges at (-3.7293, -1.4465, 0)
fillet "Abrundung3" radius 2.5 tangency weight 1.89091 1 edges at (-3.7293, -1.4465, 3)
sketch "Skizze3" plane through (0, 0, 0) normal (0, 0, -1) x (1, 0, 0)
  circle A0 centre (0, 0) radius 3.5
  circle A1 centre (0, 0) radius 2
  dimension "d24" = 4
  constraint concentric A0 A1
  measures "d24" diameter of A1
extrude "Extrusion3" add sketch "Skizze3" along normal blind 6 contours A1
thread "Gewinde1" "ISO Metric profile 4.0 M4x0.7 6g" major diameter 3.908 minor diameter 3.111 pitch 0.7 angle 60 resizes the face on face at (1.9975, 0.0997, -4)

design "M5_Stoppmutter"
Autodesk Fusion 360 part; units mm, degrees
sketch "Skizze1" plane through (0, 0, 0) normal (0, 0, 1) x (1, 0, 0)
  line L0 (4, 2.3094) -> (0, 4.6188)
  line L1 (0, 4.6188) -> (-4, 2.3094)
  line L2 (-4, 2.3094) -> (-4, -2.3094)
  line L3 (-4, -2.3094) -> (0, -4.6188)
  line L4 (0, -4.6188) -> (4, -2.3094)
  line L5 (4, -2.3094) -> (4, 2.3094)
  circle A0 centre (0, 0) radius 2.5
  dimension "d1" = 4
  dimension "d2" = 5
  constraint coincident A0.centre origin
  measures "d1" distance of A0.centre L5
  measures "d2" diameter of A0
extrude "Extrusion1" add sketch "Skizze1" along normal blind 3.2
sketch "Skizze2" plane through (0, 0, 3.2) normal (0, 0, 1) x (-1, 0, 0)
  circle A0 centre (0, 0) radius 2.5
  line L0 (-4, 2.3094) -> (-4, -2.3094)
  line L1 (-4, -2.3094) -> (0, -4.6188)
  line L2 (0, -4.6188) -> (4, -2.3094)
  line L3 (4, -2.3094) -> (4, 2.3094)
  line L4 (4, 2.3094) -> (0, 4.6188)
  line L5 (0, 4.6188) -> (-4, 2.3094)
  circle A1 centre (0, 0) radius 3.5
  constraint coincident A0.centre A1.centre
extrude "Extrusion2" add sketch "Skizze2" along normal blind 1.8 contours A1
fillet "Abrundung1" radius 0.5 1 edges at (3.2631, 1.2657, 5)
fillet "Abrundung2" radius 0.5 1 edges at (3.2631, -1.2657, 3.2)
thread "Gewinde1" "ISO Metric profile 5.0 M5x0.8 6H" major diameter 5.12 minor diameter 4.234 pitch 0.8 angle 60 resizes the face on face at (2.4876, -0.2489, 2.7333)

design "Beilagscheibe"
Autodesk Fusion 360 part; units mm, degrees
sketch "Skizze1" plane through (0, 0, 0) normal (0, 0, 1) x (1, 0, 0)
  circle A0 centre (0, 0) radius 2.65
  circle A1 centre (0, 0) radius 7.5
  dimension "d1" = 5.3
  dimension "d2" = 15
  constraint coincident A0.centre A1.centre
  constraint concentric A0 A1
  measures "d1" diameter of A0
  measures "d2" diameter of A1
extrude "Extrusion1" add sketch "Skizze1" along normal blind 1.2
fillet "Abrundung1" radius 0.2 2 edges at (-6.9925, -2.7121, 1.2) (-6.9925, -2.7121, 0)

design "M3x5"
Autodesk Fusion 360 part; units mm, degrees
sketch "Skizze1" plane through (0, 0, 0) normal (0, 0, 1) x (1, 0, 0)
  circle A0 centre (0, 0) radius 2.75
  dimension "d1" = 5.5
  constraint coincident A0.centre origin
  measures "d1" diameter of A0
extrude "Extrusion1" add sketch "Skizze1" along normal blind 3
sketch "Skizze2" plane through (0, 0, 3) normal (0, 0, 1) x (-1, 0, 0)
  circle A0 centre (0, 0) radius 2.75
  line L0 (-1.25, -0.7217) -> (0, -1.4434)
  line L1 (0, -1.4434) -> (1.25, -0.7217)
  line L2 (1.25, -0.7217) -> (1.25, 0.7217)
  line L3 (1.25, 0.7217) -> (0, 1.4434)
  line L4 (0, 1.4434) -> (-1.25, 0.7217)
  line L5 (-1.25, 0.7217) -> (-1.25, -0.7217)
  dimension "d4" = 1.25
  constraint coincident A0.centre origin
  measures "d4" distance of A0.centre L5
extrude "Extrusion2" cut sketch "Skizze2" against normal blind 1.3 contours L0 L1 L2 L3 L4 L5
sketch "Skizze3" plane through (0, 0, 0) normal (0, 0, -1) x (1, 0, 0)
  circle A0 centre (0, 0) radius 2.75
  circle A1 centre (0, 0) radius 1.5
  dimension "d7" = 3
  constraint concentric A0 A1
  measures "d7" diameter of A1
extrude "Extrusion3" add sketch "Skizze3" along normal blind 5 contours A1
thread "Gewinde1" "ISO Metric profile 3.0 M3x0.5 6g" major diameter 2.927 minor diameter 2.3555 pitch 0.5 angle 60 resizes the face on face at (1.4981, 0.0748, -3.3333)
fillet "Abrundung1" radius 0.25 2 edges at (-2.5639, -0.9944, 0) (-2.5639, -0.9944, 3)

design "Platte2" references "M5x10", "Beilagscheibe", "2020_T-Nut", "M4x6_Rundkopf+", "Zahnrad", "Platte2", "M5_Stoppmutter"
Autodesk Fusion 360 part; units mm, degrees
sketch "Skizze1" plane through (0, 0, 0) normal (1, 0, 0) x (0, 1, 0)
  line L0 (-10, 15) -> (10, 15)
  line L1 (10, 15) -> (10, -15)
  line L2 (10, -15) -> (-10, -15)
  line L3 (-10, -15) -> (-10, 15)
  circle A0 centre (0, 10) radius 2
  circle A1 centre (0, -10) radius 2
  line L4 (-9, -15) -> (-9, 15)
  line L5 (9, 15) -> (9, -15)
  dimension "d1" = 15
  dimension "d2" = 10
  dimension "d3" = 20
  dimension "d4" = 30
  dimension "d5" = 4
  dimension "d6" = 4
  dimension "d7" = 5
  dimension "d8" = 10
  dimension "d9" = 10
  dimension "d10" = 5
  dimension "d11" = 1
  dimension "d12" = 1
  constraint horizontal L0
  constraint vertical L1
  constraint horizontal L2
  constraint vertical L3
  measures "d1" distance of origin L0
  measures "d2" distance of origin L3
  measures "d3" distance of L0.start L0.end
  measures "d4" distance of L0.end L1.end
  measures "d5" diameter of A0
  measures "d6" diameter of A1
  measures "d7" distance of L2 A1.centre
  measures "d8" distance of L1 A1.centre
  measures "d9" distance of L1 A0.centre
  measures "d10" distance of L0 A0.centre
extrude "Extrusion1" add sketch "Skizze1" against normal blind 1
extrude "Extrusion2" add sketch "Skizze1" along normal blind 24 contours L0 L2 L3 L4 | L0 L1 L2 L5
chamfer "Fase1" distance 12 distance2 23 4 edges at (24, -9.5, -15) (24, 9.5, -15) (24, -9.5, 15) (24, 9.5, 15) measured on face at (24, -9.6667, 5) measured on face at (24, 9.3333, 5) measured on face at (24, -9.6667, 5) measured on face at (24, 9.3333, 5)
fillet "Abrundung1" radius 5 4 edges at (24, -9.5, -3) (24, -9.5, 3) (24, 9.5, -3) (24, 9.5, 3)
sketch "Skizze2" plane through (0, 10, 0) normal (0, 1, 0) x (-1, 0, 0)
  arc A0 (-21.2536, 4.4329) -> (-21.2536, -4.4329) centre (-18.9407, 0) ccw
  line L0 (-21.2536, -4.4329) -> (-1, -15)
  line L1 (-1, -15) -> (1, -15)
  line L2 (1, -15) -> (1, 15)
  line L3 (1, 15) -> (-1, 15)
  line L4 (-1, 15) -> (-21.2536, 4.4329)
  circle A1 centre (-18, 0) radius 2.5
  dimension "d21" = 5
  dimension "d22" = 19
  dimension "d23" = 15
  measures "d21" diameter of A1
  measures "d22" distance of L2 A1.centre
  measures "d23" vertical distance of L1.end A1.centre
extrude "Extrusion3" cut sketch "Skizze2" against normal blind 20 contours A1
fillet "Abrundung2" radius 0.5 2 edges at (0, 9, 0) (0, -9, 0)
fillet "Abrundung2" radius 1.5 2 edges at (-1, -10, 0) (-1, 10, 0)

design "Platte1"
Autodesk Fusion 360 part; units mm, degrees
sketch "Skizze1" plane through (0, 0, 0) normal (0, 0, 1) x (1, 0, 0)
  line L0 (-10, 45) -> (15, 45)
  line L1 (15, 45) -> (15, 0)
  line L2 (15, 0) -> (-10, 0)
  line L3 (-10, 0) -> (-10, 45)
  circle A0 centre (25, 39) radius 2
  line L4 (-10, 22.5) -> (15, 22.5) construction
  circle A1 centre (25, 6) radius 2
  line L5 (-10, 0) -> (-27, 0)
  line L6 (-27, 0) -> (-27, 45)
  line L7 (-27, 45) -> (-10, 45)
  line L8 (15, 45) -> (35, 45)
  line L9 (35, 45) -> (35, 0)
  line L10 (35, 0) -> (15, 0)
  line L11 (15, 0) -> (15, 45)
  circle A2 centre (11, 6.5) radius 1.5
  circle A3 centre (11, 38.5) radius 1.5
  circle A4 centre (-21, 38.5) radius 1.5
  circle A5 centre (-21, 6.5) radius 1.5
  line L12 (-27, 45) -> (-28, 45)
  line L13 (-28, 45) -> (-28, 0)
  line L14 (-28, 0) -> (-27, 0)
  line L15 (-27, 0) -> (-27, 45)
  circle A6 centre (-5, 22.5) radius 12.5
  circle A7 centre (-5, 22.5) radius 5.5 construction
  line L16 (-23, 0) -> (-23, 45) construction
  point P0 (-5, 22.5)
  dimension "d2" = 45
  dimension "d3" = 25
  dimension "d4" = 10
  dimension "d5" = 45
  dimension "d6" = 4
  dimension "d7" = 6
  dimension "d10" = 20
  dimension "d11" = 3
  dimension "d14" = 45
  dimension "d16" = 360
  dimension "d17" = 1
  dimension "d18" = 45
  dimension "d45" = 25
  dimension "d118" = 22.5
  dimension "d119" = 16
  dimension "d120" = 16
  dimension "d122" = 10
  dimension "d124" = 11
  dimension "d125" = 4
  dimension "d126" = 20
  dimension "d127" = 18
  constraint horizontal L0
  constraint vertical L1
  constraint horizontal L2
  constraint vertical L3
  constraint midpoint L3 L4.start
  constraint midpoint L1 L4.end
  constraint symmetric A0 L4 A1
  constraint perpendicular L3 L5
  constraint perpendicular L0 L6
  constraint perpendicular L3 L7
  constraint horizontal L8
  constraint vertical L9
  constraint horizontal L10
  constraint vertical L11
  constraint horizontal L12
  constraint vertical L13
  constraint horizontal L14
  constraint vertical L15
  constraint coincident P0 A6.centre
  constraint concentric A6 A7
  measures "d2" distance of L0.end L1.end
  measures "d3" distance of L0.start L0.end
  measures "d4" distance of origin L3
  measures "d5" distance of origin L0
  measures "d6" diameter of A0
  measures "d7" distance of L0 A0.centre
  measures "d10" distance of L0.end L8.end
  measures "d11" diameter of A2
  measures "d14" distance of L8.end L9.end
  measures "d17" distance of L13 L15
  measures "d18" distance of L12.end L13.end
  measures "d45" diameter of A6
  measures "d118" distance of L5 P0
  measures "d119" vertical distance of A2.centre P0
  measures "d120" horizontal distance of A2.centre P0
  measures "d122" distance of A0.centre L9
  measures "d124" diameter of A7
  measures "d126" distance of L4.end P0
  measures "d127" distance of P0 L16
extrude "Extrusion1" add sketch "Skizze1" along normal blind 1 contours L0 L1 L2 L3 L11 A6 | L3 L5 L6 L7 L15 A6 | L1 L8 L9 L10 L11 | L6 L12 L13 L14 L15
extrude "Extrusion2" add sketch "Skizze1" against normal blind 20 contours L6 L12 L13 L14 L15
sketch "Skizze2" plane through (-28, 0, 0) normal (-1, 0, 0) x (0, -1, 0)
  line L0 (-45, -20) -> (0, -20)
  line L1 (0, -20) -> (0, 1)
  line L2 (-45, 1) -> (-45, -20)
  line L3 (-39, -5) -> (-33, -5)
  line L4 (-33, -5) -> (-33, -3.5)
  line L5 (-33, -3.5) -> (-39, -3.5)
  line L6 (-39, -3.5) -> (-39, -5)
  line L7 (-22.5, 0) -> (-22.5, -20) construction
  line L8 (-22.5, -10) -> (-45, -10) construction
  line L9 (-39, -15) -> (-33, -15)
  line L10 (-33, -15) -> (-33, -16.5)
  line L11 (-33, -16.5) -> (-39, -16.5)
  line L12 (-39, -16.5) -> (-39, -15)
  line L13 (-6, -16.5) -> (-6, -15)
  line L14 (-12, -5) -> (-12, -3.5)
  line L15 (-12, -3.5) -> (-6, -3.5)
  line L16 (-12, -16.5) -> (-6, -16.5)
  line L17 (-6, -5) -> (-12, -5)
  line L18 (-22.5, -10) -> (0, -10) construction
  line L19 (-6, -3.5) -> (-6, -5)
  line L20 (-6, -15) -> (-12, -15)
  line L21 (-12, -15) -> (-12, -16.5)
  line L22 (0, 1) -> (-45, 1)
  dimension "d72" = 1.5
  dimension "d73" = 6
  dimension "d75" = 6
  dimension "d76" = 5
  constraint horizontal L3
  constraint vertical L4
  constraint horizontal L5
  constraint vertical L6
  constraint midpoint L0 L7.end
  constraint coincident L7 L8.start
  constraint coincident L2 L8.end
  constraint perpendicular L2 L8
  constraint midpoint L7 L8.start
  constraint symmetric L3.start L8 L9.start
  constraint symmetric L3.end L8 L9.end
  constraint symmetric L4.end L8 L10.end
  constraint symmetric L5.end L8 L11.end
  constraint symmetric L3.start L7 L17.start
  constraint symmetric L3.end L7 L14.start
  constraint symmetric L4.end L7 L14.end
  constraint symmetric L5.end L7 L15.end
  constraint symmetric L7 L8.start L18.start
  constraint symmetric L7 L8.end L18.end
  constraint symmetric L7 L9.start L13.end
  constraint symmetric L7 L9.end L20.end
  constraint symmetric L7 L10.end L16.start
  constraint symmetric L7 L11.end L13.start
  measures "d72" distance of L3.end L4.end
  measures "d73" distance of L4.end L5.end
  measures "d75" distance of L2 L6
  measures "d76" distance of L3 L8
extrude "Extrusion3" cut sketch "Skizze2" against normal blind 2 contours L3 L4 L5 L6 | L9 L10 L11 L12 | L13 L16 L20 L21 | L14 L15 L17 L19
extrude "Extrusion4" add 1 faces at (-27.3333, 30, -20) along direction (0, 0, -1) blind 1